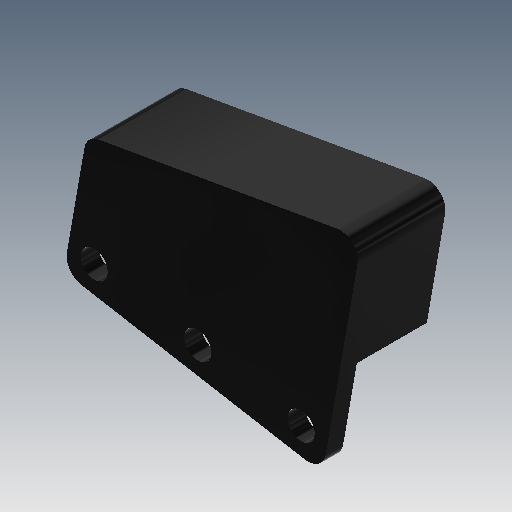
# Autodesk Inventor part: リンク_ふくらはぎ_サブフレーム_1_5
Saved by Autodesk Inventor 2017.3 (Build 213256000, 256)
## iProperties
Created: 2016-05-31
Part Number: リンク_ふくらはぎ_サブフレーム_1_5
Material: アセタール樹脂、黒
Document SubType Name: Modeling
Designer: hiroaki
Density: 1.425 g/cm^3
Appearance: 滑らか - 黒
Mass: 4.88051 g
Surface Area: 20.5902 cm^2
Volume: 3.42492 cm^3
Author: hiroaki
Autodesk Inventor part; units mm, degrees
ref_plane "YZ Plane" through (0, 0, 0) normal (1, 0, 0) x (0, 1, 0)
ref_plane "XZ Plane" through (0, 0, 0) normal (0, 1, 0) x (-1, 0, 0)
ref_plane "XY Plane" through (0, 0, 0) normal (0, 0, 1) x (1, 0, 0)
derived "下半身全体像_1_1.ipt"
sketch "スケッチ1" plane through (0, 0, 0) normal (0, 0, 1) x (1, 0, 0)
  circle A0 centre (0, 0) radius 10.5 construction
  line L0 (0, 0) -> (-12, 0) construction
  arc A1 (0, 16) -> (-12, 10.583) centre (0, 0) ccw construction
  arc A2 (-12, -10.583) -> (0, -16) centre (0, 0) ccw construction
  line L1 (0, 16) -> (39.5, 16) construction
  line L2 (39.5, 16) -> (39.5, -16) construction
  line L3 (39.5, -16) -> (0, -16) construction
  circle A3 centre (1, 13.5) radius 1.35 projected
  circle A4 centre (1, -13.5) radius 1.35 projected
  circle A5 centre (28, 13.5) radius 1.35 projected
  circle A6 centre (28, -13.5) radius 1.35 projected
  line L4 (1, 13.5) -> (1, -13.5) construction
  line L5 (1, -13.5) -> (28, -13.5) construction
  line L6 (1, 13.5) -> (28, 13.5) construction
  line L7 (28, 13.5) -> (28, -13.5) construction
  line L8 (0, 0) -> (1, 0) construction
  line L9 (32, 120) -> (32, 20) construction
  line L10 (0, 0) -> (0, 0) construction
  circle A7 centre (32, 120) radius 4.05 projected
  line L11 (0, 140) -> (0, 40) construction
  circle A8 centre (0, 40) radius 4.05 projected
  line L12 (0, 0) -> (0, -100) construction
  line L13 (32, 20) -> (32, -80) construction
  line L14 (0, 0) -> (0, 40) construction
  circle A9 centre (32, 20) radius 6.5 construction
  line L15 (32, 23.5218) -> (35.05, 21.7609) construction
  line L16 (35.05, 21.7609) -> (35.05, 18.2391) construction
  line L17 (35.05, 18.2391) -> (32, 16.4782) construction
  line L18 (32, 16.4782) -> (28.95, 18.2391) construction
  line L19 (28.95, 18.2391) -> (28.95, 21.7609) construction
  line L20 (28.95, 21.7609) -> (32, 23.5218) construction
  line L21 (21.5, 152) -> (61, 152) construction
  line L22 (61, 152) -> (61, 100.5) construction
  line L23 (61, 100.5) -> (21.5, 100.5) construction
  line L24 (21.5, 100.5) -> (21.5, 152) construction
  line L25 (21.5, 140) -> (61, 140) construction
  line L26 (16, 150.5) -> (66.5, 150.5) construction
  line L27 (66.5, 150.5) -> (66.5, 129.5) construction
  line L28 (66.5, 129.5) -> (16, 129.5) construction
  line L29 (16, 129.5) -> (16, 150.5) construction
  circle A10 centre (0, 140) radius 10.5 construction
  line L30 (-13.5, 139) -> (13.5, 139) construction
  line L31 (13.5, 139) -> (13.5, 112) construction
  line L32 (13.5, 112) -> (-13.5, 112) construction
  line L33 (-13.5, 112) -> (-13.5, 139) construction
  circle A11 centre (-13.5, 139) radius 1.35 projected
  circle A12 centre (13.5, 139) radius 1.35 projected
  circle A13 centre (-13.5, 112) radius 1.35 projected
  circle A14 centre (13.5, 112) radius 1.35 projected
  line L34 (-12, 10.583) -> (-12, -10.583) construction
  circle A15 centre (0, -100) radius 4.05 projected
  circle A16 centre (32, -80) radius 4.05 projected
  circle A17 centre (0, -100) radius 10.5 construction
  line L35 (32, -80) -> (0, -100) construction
  line L36 (45, -60.5) -> (77.5, -60.5) construction
  line L37 (77.5, -60.5) -> (77.5, -112) construction
  line L38 (77.5, -112) -> (45, -112) construction
  line L39 (45, -112) -> (45, -60.5) construction
  line L40 (45, -100) -> (77.5, -100) construction
  line L41 (39.5, -89.5) -> (83, -89.5) construction
  line L42 (83, -89.5) -> (83, -110.5) construction
  line L43 (83, -110.5) -> (39.5, -110.5) construction
  line L44 (39.5, -110.5) -> (39.5, -89.5) construction
  line L45 (1, -86.5) -> (28, -86.5) construction
  line L46 (28, -86.5) -> (28, -113.5) construction
  line L47 (28, -113.5) -> (1, -113.5) construction
  line L48 (1, -113.5) -> (1, -86.5) construction
  circle A18 centre (1, -86.5) radius 1.35 projected
  circle A19 centre (1, -113.5) radius 1.35 projected
  circle A20 centre (28, -113.5) radius 1.35 projected
  circle A21 centre (28, -86.5) radius 1.35 projected
  circle A22 centre (32, 20) radius 4.05 projected
  circle A23 centre (32, 20) radius 4.05 projected
  line L49 (10.583, 152) -> (-10.583, 152) construction
  line L50 (16, 140) -> (16, 100.5) construction
  line L51 (16, 100.5) -> (-16, 100.5) construction
  line L52 (-16, 100.5) -> (-16, 140) construction
  arc A24 (16, 140) -> (10.583, 152) centre (0, 140) ccw construction
  arc A25 (-10.583, 152) -> (-16, 140) centre (0, 140) ccw construction
  line L53 (-12, -89.417) -> (-12, -110.583) construction
  line L54 (0, -84) -> (39.5, -84) construction
  line L55 (39.5, -84) -> (39.5, -116) construction
  line L56 (39.5, -116) -> (0, -116) construction
  arc A26 (0, -84) -> (-12, -89.417) centre (0, -100) ccw construction
  arc A27 (-12, -110.583) -> (0, -116) centre (0, -100) ccw construction
  circle A28 centre (-8.5, 0) radius 1.35 projected
  circle A29 centre (0, 0) radius 8.5 construction
  line L57 (35.05, 121.7609) -> (35.05, 118.2391) construction
  line L58 (35.05, 118.2391) -> (32, 116.4782) construction
  line L59 (32, 116.4782) -> (28.95, 118.2391) construction
  line L60 (28.95, 118.2391) -> (28.95, 121.7609) construction
  line L61 (28.95, 121.7609) -> (32, 123.5218) construction
  line L62 (32, 123.5218) -> (35.05, 121.7609) construction
  line L63 (0, 152) -> (0, 140) construction
  line L64 (0, 140) -> (0, 139) construction
  line L65 (32, 20) -> (130.4808, 37.3648) construction
  line L66 (32, 20) -> (130.3245, 2.6627) construction
  line L67 (32, 20) -> (125.4678, 20) construction
  line L68 (79.2708, 11.6649) -> (80.0628, 16.1569) construction
  circle A30 centre (78.9235, 9.6953) radius 1.55
  circle A31 centre (90.7412, 7.6115) radius 1.55
  circle A32 centre (102.5589, 5.5277) radius 1.55
  line L69 (78.9235, 9.6953) -> (102.5589, 5.5277) construction
  line L70 (61.6402, 20.8662) -> (125.9068, 9.5343) construction
  line L71 (62.3878, 19.2656) -> (130.2677, 31.2347) construction
  line L72 (75.4481, 7.2618) -> (78.0517, 22.0276)
  line L73 (78.0517, 22.0276) -> (109.492, 27.5714)
  line L74 (109.492, 27.5714) -> (104.9923, 2.0523)
  line L75 (104.9923, 2.0523) -> (75.4481, 7.2618)
  line L76 (77.3582, 18.0947) -> (106.9025, 12.8852)
  point P0 (66.5, 140)
  point P1 (39.5, 0)
  point P2 (83, -100)
  point P3 (1, -100)
  point P4 (-12, -100)
  point P5 (39.5, -100)
  dimension "d1" = 20
  dimension "d2" = 10
  dimension "d3" = 48
  dimension "d4" = 2
  dimension "d5" = 3.1
  dimension "d6" = 24
  dimension "d7" = 6
  dimension "d8" = 6
  dimension "d9" = 3
  dimension "d10" = 3
  dimension "d11" = 3
  dimension "d12" = 0
  dimension "d13" = 14.9127
  dimension "d14" = 3.9936
  constraints: 24 end point, 6 point on line, 4 perpendicular, 3 centre point, 3 parallel, 2 equal radius, 2 horizontal, 1 coincident, 1 collinear, 1 equal length, 1 horizontal alignment, 1 midpoint, 1 vertical, 2 other
  measures "d1" angle of L66 L65
  measures "d2" angle of L65 L67
  measures "d3" distance from line of A22.centre L68
  measures "d4" distance from line of L66 L69.start
  measures "d5" diameter of A30
  measures "d6" distance of L69.start L69.end
  measures "d7" distance between parallel lines of L66 L70
  measures "d8" distance between parallel lines of L65 L71
  measures "d9" distance between parallel lines of L75 L69
  measures "d10" distance from line of L72 L69.start
  measures "d11" distance from line of L74 L69.end
  measures "d12" distance between parallel lines of L71 L73
  measures "d13" distance from line of L73.end L76
  measures "d14" distance of L76.start L72.end
extrude "押し出し1" add sketch "スケッチ1" against normal blind 10 contours L72 L76 L74 L75 | L72 L73 L74 L76
sketch "スケッチ3" plane through (109.492, 27.5714, -10) normal (0, 0, -1) x (-0.9848078, -0.1736482, 0)
  circle A0 centre (10.6557, -20.5048) radius 1.55 projected
  circle A1 centre (21.932, -16.4006) radius 1.55 projected
  circle A2 centre (33.2083, -12.2964) radius 1.55 projected
  line L0 (37.0534, -14.0894) -> (31.9253, 0) projected
  line L1 (0, 0) -> (8.8627, -24.35) projected
  line L2 (8.8627, -24.35) -> (37.0534, -14.0894) projected
  line L3 (33.2912, -3.7528) -> (5.1004, -14.0134)
  point P0 (112.6163, -8.1394)
  dimension "d17" = 14.9127
  dimension "d18" = 3.9936
  constraints: 2 end point, 2 point on line
  measures "d17" distance from line of L1.start L3
  measures "d18" distance of L0.end L3.start
extrude "押し出し2" cut sketch "スケッチ3" against normal blind 8
fillet "フィレット1" radius 2 4 edges at (104.9923, 2.0523, -1) (75.4481, 7.2618, -1) (109.492, 27.5714, -5) (78.0517, 22.0276, -5)
equation "\"d2\" = 0.5 * d1"
equation "\"d8\" = d7"
equation "\"d10\" = d9"
equation "\"d11\" = d10"
equation "\"d17\" = d13"
equation "\"d18\" = d14"
